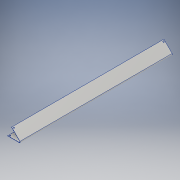
# Autodesk Inventor part: sideplate part 3
Saved by Autodesk Inventor 2018 (Build 220112000, 112)
## iProperties
Created: 2018-06-05
Part Number: sideplate part 3
Material: Aluminum 6061
Document SubType Name: Sheet Metal
Designer: John Viljoen
Density: 2.7 g/cm^3
Sheet Metal Rule: Default_mm
Appearance: Aluminum - Flat
Flat Pattern Width: 5.9677 cm
Flat Pattern Length: 36.287 cm
Flat Pattern Area: 216.55 cm^2
Sheet Metal Width: 59.67695918 mm
Sheet Metal Length: 362.87000000 mm
Sheet Metal Area: 21654.97817921 mm^2
Author: John Viljoen
Autodesk Inventor part; units mm, degrees
ref_plane "YZ Plane" through (0, 0, 0) normal (1, 0, 0) x (0, 1, 0)
ref_plane "XZ Plane" through (0, 0, 0) normal (0, 1, 0) x (-1, 0, 0)
ref_plane "XY Plane" through (0, 0, 0) normal (0, 0, 1) x (1, 0, 0)
sketch "Sketch1" plane through (0, 0, 0) normal (0, 0, 1) x (1, 0, 0)
  line L0 (0, 0) -> (27.815, 0)
  line L1 (27.815, 0) -> (27.815, 338.525)
  line L2 (27.815, 338.525) -> (0, 338.525)
  line L3 (0, 338.525) -> (0, 0)
  dimension "d0" = 27.815
  dimension "d1" = 338.525
  measures "d0" distance of L2.end L1.end
  measures "d1" distance of L1.end L0.end
extrude "Plate1" add sketch "Sketch1" along normal blind 0.5
sketch "Sketch2" plane through (28.8794, 338.525, 3.057) normal (0.7095707, 0, 0.7046342) x (0, 1, 0)
  line L0 (-338.525, 0) -> (0, 0)
  line L1 (0, 0) -> (0, 27.8153)
  line L2 (0, 27.8153) -> (-338.525, 27.8153)
  line L3 (-338.525, 27.8153) -> (-338.525, 0)
  constraints: 6 end point, 1 horizontal, 1 perpendicular, 1 vertical
edge flange "Flange1" height 32.62 angle 134.8 thickness 0.5 bend radius 1.5 thickness toward (0.7095707, 0, 0.7046342) relief straight relief width 0.5 relief depth 0.25 edges at (27.815, 169.2625, 0.5) wall of the first edge with corners at (28.8794, 0, 3.057) (28.8794, 338.525, 3.057) (9.2797, 338.525, 22.7939) (9.2797, 0, 22.7939)
bend "Bend1"
corner "Corner1"
sketch "Sketch3" plane through (9.6345, 0, 23.1462) normal (0.7095707, 0, 0.7046342) x (0.7046342, 0, -0.7095707)
  line L0 (0, 338.525) -> (27.8153, 338.525) projected
  line L1 (27.8153, 0) -> (0, 0) projected
  line L2 (0, 0) -> (3, 0) construction
  line L3 (3, 0) -> (3, 3.175) construction
  line L4 (0, 338.525) -> (3, 338.525)
  line L5 (3, 338.525) -> (3, 335.35) construction
  circle A0 centre (3, 335.35) radius 1.25
  line L6 (3, 3.175) -> (3, 3.35) construction
  circle A1 centre (3, 3.35) radius 1.25
  point P0 (9.635, 0)
  dimension "d13" = 3
  dimension "d14" = 3.175
  dimension "d16" = 3
  dimension "d17" = 3.175
  dimension "d18" = 2.5
  dimension "d34" = 0.175
  dimension "d35" = 2.5
  constraints: 10 end point, 3 coincident, 2 centre point, 2 perpendicular, 2 point on line, 1 vertical
  measures "d13" distance of L1.end L2.end
  measures "d14" distance of L2.end L3.end
  measures "d16" distance of L0.start L4.end
  measures "d17" distance of L4.end L5.end
  measures "d18" diameter of A0
  measures "d34" distance of L6.start L6.end
  measures "d35" diameter of A1
extrude "Extrusion1" cut sketch "Sketch3" against normal blind 10
sketch "Sketch4" plane through (0, 0, 0) normal (0, 0, -1) x (-1, 0, 0)
  line L0 (0, 0) -> (-27.815, 0) projected
  line L1 (0, 0) -> (-3, 0) construction
  line L2 (-3, 0) -> (-3, 3.175) construction
  line L3 (0, 338.525) -> (-3, 338.525) construction
  line L4 (0, 338.525) -> (-27.815, 338.525) construction
  line L5 (-3, 338.525) -> (-3, 335.35) construction
  circle A0 centre (-3, 335.35) radius 1.25
  line L6 (-3, 3.175) -> (-3, 3.35) construction
  circle A1 centre (-3, 3.35) radius 1.25
  dimension "d21" = 3
  dimension "d22" = 3.175
  dimension "d24" = 3
  dimension "d25" = 3.175
  dimension "d26" = 2.5
  dimension "d32" = 0.175
  dimension "d33" = 2.5
  constraints: 10 end point, 3 coincident, 2 centre point, 2 point on line, 2 vertical, 1 perpendicular
  measures "d21" distance of L0.start L1.end
  measures "d22" distance of L1.end L2.end
  measures "d24" distance of L3.start L3.end
  measures "d25" distance of L3.end L5.end
  measures "d26" diameter of A0
  measures "d32" distance of L6.start L6.end
  measures "d33" diameter of A1
extrude "Extrusion2" cut sketch "Sketch4" against normal blind 10
sketch "Sketch5" plane through (0, 0, 0) normal (0, 0, -1) x (-1, 0, 0)
  line L0 (0, 0) -> (-49.0059, 0)
  line L1 (-49.0059, 0) -> (-49.0059, 0.175)
  line L2 (-49.0059, 0.175) -> (0, 0.175)
  line L3 (0, 0.175) -> (0, 0)
  dimension "d29" = 0.175
  constraints: 8 end point, 2 parallel, 1 horizontal, 1 perpendicular
  measures "d29" distance of L0.end L1.end
extrude "Extrusion3" cut sketch "Sketch5" against normal blind 100
sketch "Sketch6" plane through (0, 338.525, 0) normal (0, 1, 0) x (1, 0, 0)
  line L0 (0, -0.5) -> (27.815, -0.5) projected
  line L1 (27.815, 0) -> (27.815, -0.5) projected
  line L2 (27.815, 0) -> (0, 0) projected
  line L3 (0, 0) -> (0, -0.5) projected
extrude "Extrusion4" add sketch "Sketch6" along normal blind 30.87
sketch "Sketch7" plane through (27.815, 338.525, 0.5) normal (0, 1, 0) x (1, 0, 0)
  line L0 (1.4191, -2.9093) -> (1.0644, -2.557) projected
  arc A0 (1.4191, -2.9093) -> (0, 0.5) centre (0, -1.5) ccw projected
  line L1 (0, 0.5) -> (0, 0) projected
  arc A1 (1.0644, -2.557) -> (0, 0) centre (0, -1.5) ccw projected
  point P0 (-27.815, 0.5)
extrude "Extrusion5" add sketch "Sketch7" along normal blind 30.87
sketch "Sketch8" plane through (9.2797, 338.525, 22.7939) normal (0, 1, 0) x (0.7095707, 0, 0.7046342)
  line L0 (0.5, 27.8153) -> (0, 27.8153) projected
  line L1 (0, 0) -> (0, 27.8153) projected
  line L2 (0, 0) -> (0.5, 0) projected
  line L3 (0.5, 0) -> (0.5, 27.8153) projected
  point P0 (-22.646, 9.635)
extrude "Extrusion6" add sketch "Sketch8" along normal blind 30.87
sketch "Sketch9" plane through (29.2341, 0.175, 3.4093) normal (0.7095707, 0, 0.7046342) x (0.7046342, 0, -0.7095707)
  circle A0 centre (-24.8153, 335.175) radius 1.25 projected
  point P0 (-18.1803, -0.175)
extrude "Extrusion7" add sketch "Sketch9" against normal up to surface (0.5 mm away)
sketch "Sketch10" plane through (0, 0, 0) normal (0, 0, -1) x (-1, 0, 0)
  circle A0 centre (-3, 335.35) radius 1.25 projected
  point P0 (0, 0)
extrude "Extrusion8" add sketch "Sketch10" against normal up to surface (0.5 mm away)
sketch "Sketch11" plane through (0, 0, 0) normal (0, 0, -1) x (-1, 0, 0)
  line L0 (0, 0.175) -> (0, 369.395) projected
  line L1 (0, 369.395) -> (0, 359.87) construction
  line L2 (0, 359.87) -> (-3.175, 359.87) construction
  circle A0 centre (-3.175, 359.87) radius 1.5
  point P0 (0, 0)
  dimension "d46" = 9.525
  dimension "d47" = 3.175
  dimension "d48" = 3
  constraints: 4 end point, 1 centre point, 1 coincident, 1 perpendicular, 1 point on line
  measures "d46" distance of L0.end L1.end
  measures "d47" distance of L1.end L2.end
  measures "d48" diameter of A0
extrude "Extrusion9" cut sketch "Sketch11" against normal blind 30.87
sketch "Sketch12" plane through (29.2341, 0.175, 3.4093) normal (0.7095707, 0, 0.7046342) x (0.7046342, 0, -0.7095707)
  line L0 (-27.8153, 0) -> (-27.8153, 369.22) projected
  line L1 (-27.8153, 369.22) -> (-27.8153, 359.695) construction
  line L2 (-27.8153, 0) -> (-27.8153, 369.22) construction
  line L3 (-27.8153, 359.695) -> (-24.6403, 359.695) construction
  circle A0 centre (-24.6403, 359.695) radius 1.5
  point P0 (-18.1803, -0.175)
  dimension "d51" = 9.525
  dimension "d52" = 3.175
  dimension "d53" = 3
  constraints: 4 end point, 1 centre point, 1 coincident, 1 perpendicular, 1 point on line
  measures "d51" distance of L0.end L1.end
  measures "d52" distance of L1.end L3.end
  measures "d53" diameter of A0
extrude "Extrusion10" cut sketch "Sketch12" against normal blind 30.87
sketch "Sketch13" plane through (0, 0, 0) normal (0, 0, -1) x (-1, 0, 0)
  line L0 (0, 369.395) -> (-53.7884, 369.395)
  line L1 (-53.7884, 369.395) -> (-53.7884, 363.045)
  line L2 (-53.7884, 363.045) -> (0, 363.045)
  line L3 (0, 363.045) -> (0, 369.395)
  point P0 (0, 0)
  dimension "d56" = 6.35
  constraints: 8 end point, 2 parallel, 1 horizontal, 1 perpendicular
  measures "d56" distance of L1.end L0.end
extrude "Extrusion11" cut sketch "Sketch13" against normal blind 30.87
equation "\"d2\" = Thickness"
equation "\"d3\" = BendReliefWidth"
equation "\"d4\" = BendReliefDepth"
equation "\"d5\" = MinimumRemnant"
equation "\"d6\" = TransitionRadius"
equation "\"d10\" = CornerReliefSize"
equation "\"d11\" = GapSize"
equation "\"d12\" = JacobiRadiusSize"
equation "\"BendRadius\" = Thickness"
equation "\"BendReliefWidth\" = Thickness"
equation "\"BendReliefDepth\" = 0.5 * Thickness"
equation "\"CornerReliefSize\" = 4 * Thickness"
equation "\"MinimumRemnant\" = 2 * Thickness"
equation "\"TransitionRadius\" = BendRadius"
equation "\"JacobiRadiusSize\" = BendRadius"
equation "\"GapSize\" = Thickness"
equation "\"Thickness\" = 0.5"
body "Solid1"
